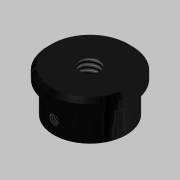
# Autodesk Inventor part: BackPair1PistonTopCap
Saved by Autodesk Inventor 2015 SP1 (Build 190203100, 203)
## iProperties
Created: 2014-09-27
Part Number: BackPair1PistonTopCap
Material: Generic
Document SubType Name: Modeling
Designer: Inventor
Density: 1 g/cm^3
Appearance: Glossy - Black
Mass: 2.07768 g
Surface Area: 12.4673 cm^2
Volume: 2.07768 cm^3
Author: Inventor
Autodesk Inventor part; units mm, degrees
ref_plane "YZ Plane" through (0, 0, 0) normal (1, 0, 0) x (0, 1, 0)
ref_plane "XY Plane" through (0, 0, 0) normal (0, 0, 1) x (1, 0, 0)
sketch "Mount" plane through (0, 0, 0) normal (0, 0, 1) x (1, 0, 0)
  circle A0 centre (0, 0) radius 9.5
  dimension "d0" = 19
  constraints: 1 centre point, 1 coincident
  measures "d0" diameter of A0
extrude "MountFeature" add sketch "Mount" along normal blind 8
sketch "Base" plane through (0, 0, 8) normal (0, 0, 1) x (1, 0, 0)
  circle A0 centre (0, 0) radius 9.5 construction
  circle A1 centre (0, 0) radius 11
  dimension "d3" = 22
  constraints: 1 centre point, 1 coincident
  measures "d3" diameter of A1
extrude "BaseFeature" add sketch "Base" along normal blind 3
chamfer "BaseChamferFeature" distance 1 angle 45 1 edges at (-11, 0, 11)
sketch "RodEndHole" plane through (0, 0, 11) normal (0, 0, 1) x (1, 0, 0)
  circle A0 centre (0, 0) radius 10 construction
hole "RodEndHoleFeature" at (0, 0, 11) direction (0, 0, -1) diameter 4.978 end through all thread size "1/4-20 UNC" class "2B" standard "ANSI Unified Screw Threads"
ref_plane "MidSidePlane" through (0, 10, 0) normal (0, 1, 0) x (-1, 0, 0)
sketch "MountHole" plane through (0, 10, 0) normal (0, 1, 0) x (-1, 0, 0)
  line L0 (-11, 8) -> (11, 8) construction
  line L1 (-9.5, 0) -> (-9.5, 8) construction
  point P0 (0, 3.5)
  dimension "d18" = 4.5
  dimension "d26" = 22
  dimension "d27" = 11
  measures "d18" distance from line of L0 point (0, 3.5)
  measures "d26" distance of L0.start L0.end
  measures "d27" horizontal distance of point (0, 3.5) L0.start
hole "MountHoleFeature" at (0, 10, 3.5) direction (0, -1, 0) diameter 2.459 end through all thread size "M3x0.5" class "6H" standard "ISO Metric profile"
equation "\"d27\" = 0.5 * d26"
